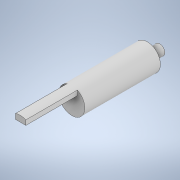
# Autodesk Inventor part: emcoder_coupler
Saved by Autodesk Inventor 2022 (Build 260153000, 153)
## iProperties
Created: 2021-12-21
Part Number: emcoder_coupler
Material: Generic
Document SubType Name: Modeling
Designer: Emazuddin Alif
Density: 1 g/cm^3
Appearance: Default
Author: Emazuddin Alif
Autodesk Inventor part; units mm, degrees
ref_plane "YZ Plane" through (0, 0, 0) normal (1, 0, 0) x (0, 1, 0)
ref_plane "XZ Plane" through (0, 0, 0) normal (0, 1, 0) x (-1, 0, 0)
ref_plane "XY Plane" through (0, 0, 0) normal (0, 0, 1) x (1, 0, 0)
sketch "Sketch1" plane through (0, 0, 0) normal (0, 0, 1) x (1, 0, 0)
  circle A0 centre (0, 0) radius 4.826
  dimension "d7" = 9.652
  constraints: 1 centre point, 1 coincident
  measures "d7" diameter of A0
extrude "Extrusion1" add sketch "Sketch1" along normal blind 27.94
sketch "Sketch2" plane through (0, 0, 27.94) normal (0, 0, 1) x (1, 0, 0)
  arc A0 (2.0632, 4.3627) -> (-1.7468, 4.4988) centre (0, 0) ccw
  circle A1 centre (0, 0) radius 4.826 projected
  line L0 (-1.7468, 4.4988) -> (-1.7468, 2.5938)
  line L1 (-1.7468, 2.5938) -> (2.0632, 2.5938)
  line L2 (2.0632, 2.5938) -> (2.0632, 4.3627)
  dimension "d8" = 3.81
  dimension "d9" = 1.905
  constraints: 6 end point, 4 point on circle, 2 perpendicular, 1 centre point, 1 coincident, 1 vertical
  measures "d8" distance of L0.end L1.end
  measures "d9" distance of L0.start L0.end
extrude "Extrusion2" add sketch "Sketch2" along normal blind 19.05 contours L2 L1 L0 A0
sketch "Sketch3" plane through (0, 0, 0) normal (0, 0, -1) x (-1, 0, 0)
  circle A0 centre (0, 0) radius 1.905
  dimension "d6" = 3.81
  constraints: 1 centre point, 1 coincident
  measures "d6" diameter of A0
extrude "Extrusion3" add sketch "Sketch3" along normal blind 4.572
body "Solid1"
